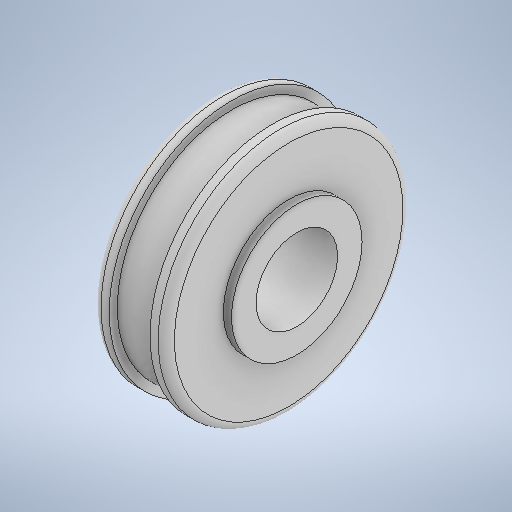
# Autodesk Inventor part: 11 base
Saved by Autodesk Inventor 2025.1 (Build 291241000, 241)
## iProperties
Created: 2024-09-12
Part Number: 11 base
Material: Generisch
Document SubType Name: Modeling
Designer: ffogue
Density: 1 g/cm^3
Appearance: Vorgabe
Author: ffogue
Autodesk Inventor part; units mm, degrees
ref_plane "YZ Plane" through (0, 0, 0) normal (1, 0, 0) x (0, 1, 0)
ref_plane "XZ Plane" through (0, 0, 0) normal (0, 1, 0) x (-1, 0, 0)
ref_plane "XY Plane" through (0, 0, 0) normal (0, 0, 1) x (1, 0, 0)
sketch "Sketch1" plane through (0, 0, 0) normal (0, 0, 1) x (1, 0, 0)
  line L0 (-4.5, 0) -> (-4.5, 15)
  line L1 (-4.5, 15) -> (-2.5, 15)
  line L2 (-2.5, 15) -> (-2.5, 14)
  line L3 (-2.5, 14) -> (2.5, 14)
  line L4 (2.5, 14) -> (2.5, 15)
  line L5 (2.5, 15) -> (4.5, 15)
  line L6 (4.5, 15) -> (4.5, 0)
  line L7 (4.5, 0) -> (-4.5, 0)
  line L8 (4.5, 8) -> (5.5, 8)
  line L9 (5.5, 8) -> (5.5, 0)
  line L10 (4.5, 0) -> (5.5, 0)
  line L11 (0, 14) -> (0, 0) construction
  dimension "d0" = 30
  dimension "d1" = 2
  dimension "d2" = 2
  dimension "d3" = 9
  dimension "d4" = 16
  dimension "d5" = 1
  dimension "d6" = 28
  constraints: 24 end point, 9 perpendicular, 3 point on line, 1 horizontal, 1 midpoint, 1 vertical, 1 vertical alignment
  measures "d0" diameter of L5 L7
  measures "d1" distance of L4.end L5.end
  measures "d2" distance of L0.end L1.end
  measures "d3" distance between parallel lines of L6 L0
  measures "d4" diameter of L8 L10
  measures "d5" distance of L8.start L8.end
  measures "d6" diameter of L3 L7
revolve "Revolution1" add sketch "Sketch1" angle 360 about axis through (4.5, 0, 0) along (-1, 0, 0)
sketch "Sketch3" plane through (-4.5, 0, 0) normal (-1, 0, 0) x (0, 0, 1)
  circle A0 centre (0, 0) radius 15 projected
  point P0 (0, 0)
  constraints: 1 coincident
hole "Hole2" at (-4.5, 0, 0) direction (1, 0, 0) diameter 4.134 depth 10 thread size "M5x0.8" class "6H" standard "ISO Metric profile"
sketch "Sketch4" plane through (5.5, 0, 0) normal (1, 0, 0) x (0, 0, -1)
  circle A0 centre (0, 0) radius 8 projected
  point P0 (0, 0)
  constraints: 1 coincident
hole "Hole3" at (5.5, 0, 0) direction (-1, 0, 0) diameter 10 depth 9
fillet "Fillet2" radius 1 2 edges at (-4.5, -15, 0) (4.5, -15, 0)
body "Solid1"
